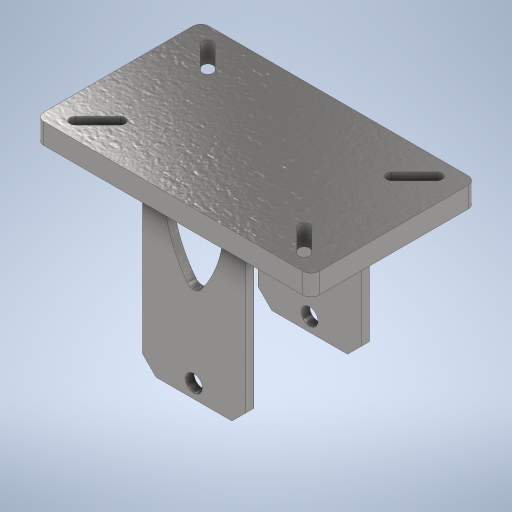
# Autodesk Inventor part: Koerper
Saved by Autodesk Inventor 2024 (Build 280153000, 153)
## iProperties
Created: 2024-02-12
Part Number: Koerper
Material: Stahl, galvanisiert
Document SubType Name: Modeling
Designer: ffogue
Density: 7.85 g/cm^3
Appearance: Galvanisiert
Author: ffogue
Autodesk Inventor part; units mm, degrees
ref_plane "YZ Plane" through (0, 0, 0) normal (1, 0, 0) x (0, 1, 0)
sketch "Skizze1" plane through (0, 0, 0) normal (0, 0, 1) x (1, 0, 0)
  line L0 (0, 0) -> (20, 0)
  line L1 (20, 0) -> (20, 12)
  line L2 (20, 12) -> (0, 12)
  line L3 (0, 12) -> (0, 0)
  point P0 (0, 6)
  dimension "d0" = 20
  dimension "d1" = 12
  constraints: 8 end point, 2 parallel, 1 horizontal, 1 midpoint, 1 perpendicular
  measures "d0" distance from line of L1 point (0, 6)
  measures "d1" distance between parallel lines of L0 L2
extrude "Extrusion1" add sketch "Skizze1" along normal blind 1.5
sketch "Skizze2" plane through (0, 0, 1.5) normal (0, 0, 1) x (1, 0, 0)
  line L0 (1.6868, 10.8132) -> (3.3132, 9.1868) construction
  line L1 (1.4217, 10.548) -> (3.048, 8.9217)
  line L2 (3.5783, 9.452) -> (1.952, 11.0783)
  arc A0 (1.952, 11.0783) -> (1.4217, 10.548) centre (1.6868, 10.8132) ccw
  arc A1 (3.048, 8.9217) -> (3.5783, 9.452) centre (3.3132, 9.1868) ccw
  line L3 (0, 12) -> (0, 0) projected
  line L4 (18.3132, 10.8132) -> (16.6868, 9.1868) construction
  line L5 (18.5783, 10.548) -> (16.952, 8.9217)
  line L6 (16.4217, 9.452) -> (18.048, 11.0783)
  arc A2 (18.5783, 10.548) -> (18.048, 11.0783) centre (18.3132, 10.8132) ccw
  arc A3 (16.4217, 9.452) -> (16.952, 8.9217) centre (16.6868, 9.1868) ccw
  line L7 (20, 0) -> (20, 12) projected
  line L8 (0, 0) -> (20, 0) projected
  line L9 (10, 0) -> (10, 12) construction
  line L10 (20, 12) -> (0, 12) projected
  point P0 (2.5, 10)
  point P1 (17.5, 10)
  dimension "d7" = 15
  dimension "d8" = 7.5
  dimension "d9" = 0.75
  dimension "d10" = 2
  dimension "d11" = 2.3
  dimension "d12" = 45
  constraints: 18 end point, 8 point on circle, 8 tangent, 4 centre point, 3 midpoint, 2 horizontal alignment, 2 parallel, 1 equal radius, 1 perpendicular, 1 vertical
  measures "d7" distance of point (17.5, 10) point (2.5, 10)
  measures "d8" distance from line of L9 point (2.5, 10)
  measures "d9" distance between parallel lines of L2 L1
  measures "d10" distance from line of L10 point (2.5, 10)
  measures "d11" distance of L2.start L2.end
  measures "d12" angle of L3 L1
extrude "Extrusion2" cut sketch "Skizze2" against normal up to surface (1.5 mm away) contours A0 L2 A1 L1 | L5 A3 L6 A2
ref_plane "Arbeitsebene1" through (0, 6, 0) normal (0, 1, 0) x (-1, 0, 0)
mirror "Spiegeln1" about plane through (0, 6, 0) normal (0, 1, 0) of "Extrusion2"
sketch "Skizze3" plane through (0, 0, 0) normal (0, 0, -1) x (-1, 0, 0)
  line L0 (-20, 12) -> (0, 12) projected
  line L1 (-10, 12) -> (-10, 0) construction
  line L2 (0, 0) -> (-20, 0) projected
  line L3 (-6.25, 10.5) -> (-13.75, 10.5)
  line L4 (-13.75, 10.5) -> (-13.75, 9.9)
  line L5 (-13.75, 9.9) -> (-6.25, 9.9)
  line L6 (-6.25, 9.9) -> (-6.25, 10.5)
  dimension "d16" = 1.5
  dimension "d17" = 7.5
  dimension "d18" = 0.6
  constraints: 10 end point, 2 midpoint, 2 parallel, 1 horizontal, 1 perpendicular, 1 other
  measures "d16" distance between parallel lines of L3 L0
  measures "d17" distance between parallel lines of L4 L6
  measures "d18" distance between parallel lines of L5 L3
extrude "Extrusion3" add sketch "Skizze3" along normal blind 12
chamfer "Fasen1" distance 1 angle 45 2 edges at (13.75, 10.2, -12) (6.25, 10.2, -12)
sketch "Skizze4" plane through (6.25, 10.5, 0) normal (0, 1, 0) x (1, 0, 0)
  line L0 (7.5, 0) -> (0, 0) projected
  line L1 (3.75, 0) -> (3.75, 5.4569) construction
  arc A0 (5.9, 0) -> (3.75, 5.4569) centre (-2.1, 0) ccw
  arc A1 (3.75, 5.4569) -> (1.6, 0) centre (9.6, 0) ccw
  line L2 (13.75, 0) -> (-6.25, 0) projected
  line L3 (7.5, 0) -> (7.5, 11) projected
  dimension "d24" = 8
  dimension "d25" = 1.6
  constraints: 4 point on circle, 3 point on line, 2 centre point, 2 end point, 1 equal radius, 1 horizontal alignment, 1 midpoint, 1 vertical
  measures "d24" radius of A0
  measures "d25" distance from line of L3 A0.start
extrude "Extrusion4" cut sketch "Skizze4" against normal up to surface (0.6 mm away)
fillet "Rundung1" radius 0.6 1 edges at (10, 10.2, -5.4569)
sketch "Skizze5" plane through (7.25, 10.5, -12) normal (0, 1, 0) x (1, 0, 0)
  circle A0 centre (2.75, -1) radius 0.6
  line L0 (0, 0) -> (5.5, 0) projected
  line L1 (-1, -12) -> (-1, -1) projected
  point P0 (-7.25, -12)
  point P1 (2.75, 0)
  dimension "d30" = 1
  dimension "d31" = 1.2
  constraints: 1 centre point, 1 midpoint, 1 vertical alignment
  measures "d30" distance of point (2.75, 0) A0.centre
  measures "d31" diameter of A0
extrude "Extrusion5" cut sketch "Skizze5" against normal up to surface (0.6 mm away)
ref_plane "Arbeitsebene2" through (0, 6, 0) normal (0, 1, 0) x (-1, 0, 0)
mirror "Spiegeln2" about plane through (0, 6, 0) normal (0, 1, 0) of "Extrusion3", "Extrusion4", "Extrusion5", "Fasen1", "Rundung1"
fillet "Rundung2" radius 0.6 4 edges at (20, 12, 0.75) (0, 12, 0.75) (0, 0, 0.75) (20, 0, 0.75)
